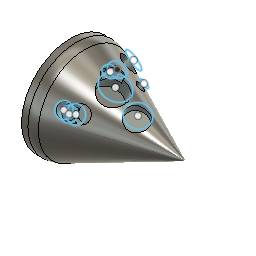
Aguja Daños Esfera v1 (Autodesk Fusion 360 design; units mm, degrees)
Autodesk Fusion 360 part; units mm, degrees
sketch "Sketch1" plane through (0, 0, 0) normal (0, 1, 0) x (1, 0, 0)
  line L0 (0, 0) -> (272, 0)
  line L1 (0, 0) -> (0, -115)
  line L2 (0, -115) -> (14.7579, -115)
  line L3 (35.0449, -110.5022) -> (272, 0)
  arc A0 (14.7579, -115) -> (35.0449, -110.5022) centre (14.7579, -67) ccw
  point P0 (25.4, -115)
  dimension "d1" = 272
  dimension "d2" = 115
  dimension "d3" = 25.4
  dimension "d4" = 48
  constraint coincident L0.start L1.start
  constraint horizontal L0
  constraint perpendicular L0 L1
  constraint perpendicular L1 L2
  constraint coincident P0 L2
  constraint coincident P0 L3
  constraint tangent L2 A0
  constraint tangent L3 A0
  measures "d1" distance of L0.start L0.end
  measures "d2" distance of L0.start L1.end
  measures "d3" distance of L1.end P0
  measures "d4" radius of A0
revolve "Revolve1" add sketch "Sketch1" angle 360 about axis through (0, 0, 0) along (1, 0, 0)
ref_plane "WorkPlane1" through (153.5224, 55.2511, 0) normal (0.422644, 0.906296, 0) x (0, 0, 1)
sketch "Sketch2" plane through (153.5224, 55.2511, 0) normal (0.422644, 0.906296, 0) x (0, 0, 1)
  circle A0 through (14.3481, -70.4275, 10) (-7.2623, -57.9507, 10) (-7.2623, -82.9042, 10)
  circle A1 through (3.3534, -67.3663, 10) (-22.8818, -52.2194, 10) (-22.8818, -82.5132, 10)
  circle A2 through (42.8899, -42.1316, 8.2951) (-2.7991, -15.7531, 8.2951) (-2.7991, -68.5102, 8.2951)
  circle A3 through (-41.0456, -28.229, -2.2785) (-54.247, -19.7655, -12.298) (-54.247, -38.3037, -10.6761)
  circle A4 through (-57.6778, -77.6745, -4.9196) (-80.3204, -59.3249, -28.1428) (-84.48, -96.0242, -23.1856)
  circle A5 through (100.4939, -69.9513, -49.6405) (83.5135, -56.0868, -32.6601) (83.5135, -83.8157, -32.6601)
  circle A6 through (97.2708, -59.3404, -49.0121) (81.4225, -46.4004, -33.1639) (81.4225, -72.2804, -33.1639)
  circle A7 through (97.0928, -47.6685, -39.3685) (81.7151, -32.1896, -17.407) (81.7151, -63.1473, -17.407)
  circle A8 through (40.3849, 21.2097, 0.8891) (4.3103, 42.772, 10.5552) (4.3103, -0.3527, 10.5552)
extrude "Extrude1" cut sketch "Sketch2" against normal blind 40 contours A2 in plane through (157.0283, 62.7689, 0) normal (0.422644, 0.906296, 0)
extrude "Extrude2" cut sketch "Sketch2" against normal blind 20 contours A0 A1 | A0 A1 | A0 A1 in plane through (157.7489, 64.3141, 0) normal (0.422644, 0.906296, 0)
extrude "Extrude3" cut sketch "Sketch2" against normal blind 30 contours A8 in plane through (158.1401, 65.1531, 2.9275) normal (0.408243, 0.875414, 0.258819)
extrude "Extrude4" cut sketch "Sketch2" against normal blind 20 contours A3 in plane through (161.5784, 69.2035, -11.2811) normal (0.409596, 0.709395, -0.573576)
extrude "Extrude5" cut sketch "Sketch2" against normal blind 50 contours A4 in plane through (162.7192, 67.0376, -12.2249) normal (0.476222, 0.610324, -0.633022)
extrude "Extrude6" cut sketch "Sketch2" against normal blind 20 contours A7 in plane through (167.3289, 84.8569, 46.6531) normal (0.242419, 0.51983, 0.819152)
extrude "Extrude7" cut sketch "Sketch2" against normal blind 40 contours A5 in plane through (164.2689, 78.2952, 25.4267) normal (0.298854, 0.640848, 0.707107)
extrude "Extrude8" cut sketch "Sketch2" against normal blind 20 contours A6 in plane through (163.7205, 77.1194, 24.1293) normal (0.298854, 0.640848, 0.707107)
extrude "Extrude9" cut sketch "Sketch2" against normal blind 50 contours A7 in plane through (167.3289, 84.8569, 46.6531) normal (0.242419, 0.51983, 0.819152)
